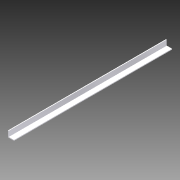
# Autodesk Inventor part: angle support
Saved by Autodesk Inventor 2012 (Build 160160000, 160)
## iProperties
Created: 2013-05-09
Part Number: angle support
Material: Default
Document SubType Name: Modeling
Designer: Fabian
Density: 1 g/cm^3
Author: Fabian
Autodesk Inventor part; units mm, degrees
ref_plane "YZ Plane" through (0, 0, 0) normal (1, 0, 0) x (0, 1, 0)
ref_plane "XZ Plane" through (0, 0, 0) normal (0, 1, 0) x (-1, 0, 0)
ref_plane "XY Plane" through (0, 0, 0) normal (0, 0, 1) x (1, 0, 0)
sketch "Sketch1" plane through (0, 0, 0) normal (0, 0, 1) x (1, 0, 0)
  line L0 (-8.3916, 29.4986) -> (-3.6291, 29.4986)
  line L1 (-3.6291, 29.4986) -> (-3.6291, -8.6014)
  line L2 (-3.6291, -8.6014) -> (-8.3916, -8.6014)
  line L3 (-8.3916, -8.6014) -> (-8.3916, 29.4986)
  line L4 (-3.6291, -8.6014) -> (29.7084, -8.6014)
  line L5 (29.7084, -8.6014) -> (29.7084, -3.8389)
  line L6 (29.7084, -3.8389) -> (-3.6291, -3.8389)
  line L7 (-3.6291, -3.8389) -> (-3.6291, -8.6014)
  point P0 (0, 0)
  dimension "d0" = 38.1
  dimension "d1" = 38.1
  dimension "d2" = 4.7625
  dimension "d3" = 4.7625
  constraints: 16 end point, 4 parallel, 2 horizontal, 2 perpendicular
  measures "d0" distance between parallel lines of L5 L3
  measures "d1" distance of L2.end L0.start
  measures "d2" distance between parallel lines of L3 L1
  measures "d3" distance between parallel lines of L6 L4
extrude "Extrusion1" add sketch "Sketch1" along normal blind 1000
body "Solid1"
